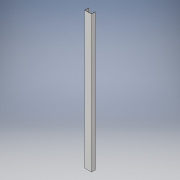
# Autodesk Inventor part: Grundstange Bauhaus
Saved by Autodesk Inventor 2017 (Build 210142000, 142)
## iProperties
Part Number: Grundstange Bauhaus
Material: Generisch
Document SubType Name: Modeling
Designer: pgmadmin
Density: 1 g/cm^3
Appearance: Vorgabe
Author: pgmadmin
Autodesk Inventor part; units mm, degrees
ref_plane "YZ Plane" through (0, 0, 0) normal (1, 0, 0) x (0, 1, 0)
ref_plane "XZ Plane" through (0, 0, 0) normal (0, 1, 0) x (-1, 0, 0)
ref_plane "XY Plane" through (0, 0, 0) normal (0, 0, 1) x (1, 0, 0)
sketch "Skizze1" plane through (0, 0, 0) normal (0, 0, 1) x (1, 0, 0)
  line L0 (-25.9341, 8.8004) -> (-25.9341, -10.6996)
  line L1 (-25.9341, -10.6996) -> (9.5659, -10.6996)
  line L2 (9.5659, -10.6996) -> (9.5659, 8.8004)
  line L3 (9.5659, 8.8004) -> (8.0659, 8.8004)
  line L4 (8.0659, 8.8004) -> (8.0659, -9.1996)
  line L5 (8.0659, -9.1996) -> (-24.4341, -9.1996)
  line L6 (-24.4341, -9.1996) -> (-24.4341, 8.8004)
  line L7 (-24.4341, 8.8004) -> (-25.9341, 8.8004)
  point P0 (0, 0)
  dimension "d0" = 35.5
  dimension "d1" = 32.5
  dimension "d2" = 1.5
  dimension "d3" = 19.5
  dimension "d4" = 1.5
  constraints: 16 end point, 7 perpendicular, 1 point on line, 1 vertical
  measures "d0" distance between parallel lines of L2 L0
  measures "d1" distance between parallel lines of L4 L6
  measures "d2" distance between parallel lines of L0 L6
  measures "d3" distance between parallel lines of L3 L1
  measures "d4" distance between parallel lines of L1 L5
extrude "Extrusion1" add sketch "Skizze1" along normal blind 700
